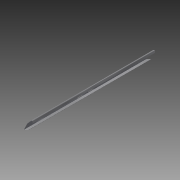
# Autodesk Inventor part: 2in rail right
Saved by Autodesk Inventor 2015 SP1 (Build 190203100, 203)
## iProperties
Created: 2015-01-12
Part Number: 2in rail right
Material: Steel, Alloy
Document SubType Name: Modeling
Designer: Jarod
Density: 7.73 g/cm^3
Appearance: Semi-Polished
Author: Jarod
Autodesk Inventor part; units mm, degrees
ref_plane "YZ Plane" through (0, 0, 0) normal (1, 0, 0) x (0, 1, 0)
ref_plane "XZ Plane" through (0, 0, 0) normal (0, 1, 0) x (-1, 0, 0)
ref_plane "XY Plane" through (0, 0, 0) normal (0, 0, 1) x (1, 0, 0)
sketch "Sketch1" plane through (0, 0, 0) normal (0, 0, 1) x (1, 0, 0)
  line L0 (0, 0) -> (-12.7, 0) construction
  line L1 (-12.7, 0) -> (-12.7, 53.975) construction
  line L2 (-12.7, 53.975) -> (0, 53.975) construction
  line L3 (0, 53.975) -> (0, 0) construction
  line L4 (-12.7, 53.975) -> (-25.4, 53.975) construction
  line L5 (-12.7, 53.975) -> (0, 53.975) construction
  line L6 (-25.4, 53.975) -> (-25.4, 0) construction
  line L7 (-25.4, 0) -> (-12.7, 0) construction
  circle A0 centre (-12.7, 6.35) radius 6.35 construction
  circle A1 centre (-12.7, 47.625) radius 6.35 construction
  line L8 (-12.7, 47.625) -> (-18.1993, 50.8) construction
  line L9 (-12.7, 47.625) -> (-6.35, 47.625) construction
  line L10 (-12.7, 47.625) -> (-7.2007, 50.8) construction
  line L11 (-12.7, 47.625) -> (-6.35, 47.625) construction
  line L12 (0, 0) -> (-25.4, 0)
  line L13 (0, 0) -> (0, -1.5875)
  line L14 (0, 0) -> (1.5875, 0) construction
  line L15 (0, -1.5875) -> (-26.9875, -1.5875)
  arc A2 (-7.2007, 50.8) -> (-18.1993, 50.8) centre (-12.7, 47.625) ccw
  line L16 (-7.2007, 50.8) -> (0, 38.328)
  line L17 (-7.2007, 50.8) -> (7.2007, 50.8) construction
  line L18 (-18.1993, 50.8) -> (-24.5493, 39.8015)
  line L19 (-18.1993, 50.8) -> (-5.4993, 50.8) construction
  line L20 (-25.4, 0) -> (-25.4, 36.6265)
  line L21 (-19.5741, 51.5937) -> (-26.1368, 40.2268)
  line L22 (-26.9875, -1.5875) -> (-26.9875, 37.0518)
  arc A3 (-26.1368, 40.2268) -> (-26.9875, 37.0518) centre (-20.6375, 37.0518) ccw
  arc A4 (-24.5493, 39.8015) -> (-25.4, 36.6265) centre (-19.05, 36.6265) ccw
  line L23 (-5.8259, 51.5937) -> (1.3748, 39.1217)
  arc A5 (-5.8259, 51.5937) -> (-19.5741, 51.5937) centre (-12.7, 47.625) ccw
  arc A6 (0, 38.328) -> (1.3748, 39.1217) centre (0.6874, 38.7248) ccw
  point P0 (-25.4, 38.328)
  dimension "d0" = 12.7
  dimension "d1" = 53.975
  dimension "d2" = 12.7
  dimension "d3" = 180
  dimension "d4" = 53.975
  dimension "d5" = 90
  dimension "d6" = 12.7
  dimension "d7" = 12.7
  dimension "d8" = 6.35
  dimension "d9" = 6.35
  dimension "d10" = 6.35
  dimension "d11" = 150
  dimension "d12" = 6.35
  dimension "d13" = 30
  dimension "d14" = 1.5875
  dimension "d15" = 90
  dimension "d16" = 26.9875
  dimension "d17" = 6.35
  dimension "d18" = 60
  dimension "d19" = 120
  dimension "d20" = 90
  dimension "d21" = 1.5875
  dimension "d22" = 6.35
  dimension "d23" = 6.35
  dimension "d24" = 1.5875
  dimension "d25" = 7.9375
  dimension "d26" = 0
  constraints: 48 end point, 10 point on circle, 8 horizontal, 7 centre point, 6 equal length, 6 point on line, 6 tangent, 4 parallel, 3 perpendicular, 2 vertical
  measures "d0" distance of L1.end L2.end
  measures "d1" distance of L0.end L1.end
  measures "d2" distance of L1.end L4.end
  measures "d3" angle of L4 L5
  measures "d4" distance of L4.end L6.end
  measures "d5" angle of L6 L4
  measures "d6" diameter of A0
  measures "d7" diameter of A1
  measures "d8" distance from line of L0 A0.centre
  measures "d9" distance from line of L2 L8.start
  measures "d10" distance of L8.start L8.end
  measures "d11" angle of L9 L8
  measures "d12" distance of L8.start L10.end
  measures "d13" angle of L11 L10
  measures "d14" distance of L0.start L13.end
  measures "d15" angle of L13 L14
  measures "d16" distance of L13.end L15.end
  measures "d17" radius of A2
  measures "d18" angle of L16 L17
  measures "d19" angle of L18 L19
  measures "d20" angle of L15 L22
  measures "d21" distance between parallel lines of L21 L18
  measures "d22" radius of A3
  measures "d23" radius of A4
  measures "d24" distance between parallel lines of L16 L23
  measures "d25" radius of A5
  measures "d26" distance of L8.start A5.centre
extrude "Extrusion1" add sketch "Sketch1" along normal blind 1689.1
sketch "Sketch2" plane through (-26.9875, -1.5875, 0) normal (-1, 0, 0) x (0, 0, 1)
  line L0 (0, 38.6393) -> (0, 0) projected
  line L1 (0, 0) -> (1689.1, 0) projected
  line L2 (1689.1, 38.6393) -> (1689.1, 0) projected
  line L3 (0, 38.6393) -> (1689.1, 38.6393) projected
  point P0 (0, 1.5875)
  point P1 (1651, 19.05)
  dimension "d29" = 19.05
  dimension "d30" = 38.1
  measures "d29" distance from line of point (1651, 19.05) L1
  measures "d30" distance from line of point (1651, 19.05) L2
hole "Hole1" at (-26.9875, 17.4625, 1651) direction (1, 0, 0) diameter 9.525 end through all
sketch "Sketch3" plane through (-26.9875, -1.5875, 0) normal (-1, 0, 0) x (0, 0, 1)
  circle A0 centre (1651, 19.05) radius 4.7625 projected
  line L0 (0, 38.6393) -> (0, 0) projected
  line L1 (0, 0) -> (1689.1, 0) projected
  line L2 (1689.1, 38.6393) -> (1689.1, 0) projected
  line L3 (0, 38.6393) -> (1689.1, 38.6393) projected
  circle A1 centre (31.75, 19.05) radius 4.7625
  line L4 (15.875, 28.575) -> (15.875, 25.4) construction
  line L5 (15.875, 28.575) -> (15.875, 31.75) construction
  line L6 (12.7, 28.575) -> (12.7, 31.75) construction
  line L7 (12.7, 28.575) -> (12.7, 25.4) construction
  line L8 (15.875, 12.7) -> (15.875, 15.875) construction
  line L9 (12.7, 12.7) -> (12.7, 15.875) construction
  line L10 (15.875, 12.7) -> (15.875, 9.525) construction
  line L11 (12.7, 12.7) -> (12.7, 9.525) construction
  arc A2 (15.875, 25.4) -> (15.875, 31.75) centre (15.875, 28.575) ccw
  arc A3 (12.7, 31.75) -> (12.7, 25.4) centre (12.7, 28.575) ccw
  arc A4 (15.875, 9.525) -> (15.875, 15.875) centre (15.875, 12.7) ccw
  arc A5 (12.7, 15.875) -> (12.7, 9.525) centre (12.7, 12.7) ccw
  line L12 (15.875, 31.75) -> (12.7, 31.75)
  line L13 (15.875, 25.4) -> (12.7, 25.4)
  line L14 (15.875, 15.875) -> (12.7, 15.875)
  line L15 (15.875, 9.525) -> (12.7, 9.525)
  point P0 (0, 1.5875)
  dimension "d45" = 12.7
  dimension "d46" = 15.875
  dimension "d47" = 31.75
  dimension "d48" = 12.7
  dimension "d49" = 15.875
  dimension "d50" = 9.525
  dimension "d51" = 19.05
  dimension "d52" = 12.7
  dimension "d53" = 12.7
  dimension "d54" = 28.575
  dimension "d55" = 28.575
  dimension "d56" = 3.175
  dimension "d57" = 3.175
  dimension "d58" = 3.175
  dimension "d59" = 3.175
  dimension "d60" = 3.175
  dimension "d61" = 3.175
  dimension "d62" = 3.175
  dimension "d63" = 3.175
  dimension "d64" = 3.175
  dimension "d65" = 3.175
  dimension "d66" = 3.175
  dimension "d67" = 3.175
  constraints: 24 end point, 8 point on circle, 8 vertical, 5 centre point, 1 coincident
  measures "d45" distance from line of L0 L6.start
  measures "d46" distance from line of L0 L4.start
  measures "d47" distance from line of L0 point (31.75, 19.05)
  measures "d48" distance from line of L0 L9.start
  measures "d49" distance from line of L0 L8.start
  measures "d50" diameter of A1
  measures "d51" distance from line of L1 A1.centre
  measures "d52" distance from line of L9.start L1
  measures "d53" distance from line of L1 L8.start
  measures "d54" distance from line of L6.start L1
  measures "d55" distance from line of L4.start L1
  measures "d56" distance of L4.start L4.end
  measures "d57" distance of L4.start L5.end
  measures "d58" distance of L6.start L6.end
  measures "d59" distance of L6.start L7.end
  measures "d60" distance of L8.start L8.end
  measures "d61" distance of L9.start L9.end
  measures "d62" distance of L8.start L10.end
  measures "d63" distance of L9.start L11.end
  measures "d64" radius of A2
  measures "d65" radius of A3
  measures "d66" radius of A4
  measures "d67" radius of A5
extrude "Extrusion2" cut sketch "Sketch3" against normal blind 25.4 contours A1 | L13 A3 L12 A2 | L15 A5 L14 A4
sketch "Sketch4" plane through (-26.9875, -1.5875, 0) normal (-1, 0, 0) x (0, 0, 1)
  line L0 (12.7, 15.875) -> (15.875, 15.875) projected
  arc A0 (15.875, 9.525) -> (15.875, 15.875) centre (15.875, 12.7) ccw projected
  line L1 (15.875, 9.525) -> (12.7, 9.525) projected
  arc A1 (12.7, 15.875) -> (12.7, 9.525) centre (12.7, 12.7) ccw projected
  line L2 (12.7, 31.75) -> (15.875, 31.75) projected
  arc A2 (15.875, 25.4) -> (15.875, 31.75) centre (15.875, 28.575) ccw projected
  line L3 (15.875, 25.4) -> (12.7, 25.4) projected
  arc A3 (12.7, 31.75) -> (12.7, 25.4) centre (12.7, 28.575) ccw projected
  circle A4 centre (31.75, 19.05) radius 4.7625 projected
  circle A5 centre (1651, 19.05) radius 4.7625 projected
  line L4 (0, 38.6393) -> (0, 0) projected
  line L5 (0, 0) -> (1689.1, 0) projected
  line L6 (1689.1, 38.6393) -> (1689.1, 0) projected
  line L7 (0, 38.6393) -> (1689.1, 38.6393) projected
  point P0 (0, 1.5875)
  point P1 (101.6, 25.4)
  point P2 (88.9, 12.7)
  point P3 (76.2, 25.4)
  point P4 (63.5, 12.7)
  dimension "d70" = 63.5
  dimension "d71" = 76.2
  dimension "d72" = 88.9
  dimension "d73" = 101.6
  dimension "d74" = 12.7
  dimension "d77" = 12.7
  dimension "d120" = 25.4
  dimension "d121" = 25.4
  measures "d70" distance from line of L4 point (63.5, 12.7)
  measures "d71" distance from line of L4 point (76.2, 25.4)
  measures "d72" distance from line of L4 point (88.9, 12.7)
  measures "d73" distance from line of L4 point (101.6, 25.4)
  measures "d74" distance from line of L5 point (63.5, 12.7)
  measures "d77" distance from line of L5 point (88.9, 12.7)
  measures "d120" distance from line of point (76.2, 25.4) L5
  measures "d121" distance from line of L5 point (101.6, 25.4)
hole "Hole2" at (-26.9875, 23.8125, 101.6) at (-26.9875, 11.1125, 88.9) at (-26.9875, 23.8125, 76.2) at (-26.9875, 11.1125, 63.5) direction (1, 0, 0) diameter 6.35 end through all
sketch "Sketch6" plane through (-26.9875, -1.5875, 0) normal (-1, 0, 0) x (0, 0, 1)
  circle A0 centre (76.2, 25.4) radius 3.175 projected
  circle A1 centre (101.6, 25.4) radius 3.175 projected
  circle A2 centre (88.9, 12.7) radius 3.175 projected
  circle A3 centre (63.5, 12.7) radius 3.175 projected
  line L0 (12.7, 15.875) -> (15.875, 15.875) projected
  arc A4 (15.875, 9.525) -> (15.875, 15.875) centre (15.875, 12.7) ccw projected
  line L1 (15.875, 9.525) -> (12.7, 9.525) projected
  arc A5 (12.7, 15.875) -> (12.7, 9.525) centre (12.7, 12.7) ccw projected
  line L2 (12.7, 31.75) -> (15.875, 31.75) projected
  arc A6 (15.875, 25.4) -> (15.875, 31.75) centre (15.875, 28.575) ccw projected
  line L3 (15.875, 25.4) -> (12.7, 25.4) projected
  arc A7 (12.7, 31.75) -> (12.7, 25.4) centre (12.7, 28.575) ccw projected
  circle A8 centre (31.75, 19.05) radius 4.7625 projected
  circle A9 centre (1651, 19.05) radius 4.7625 projected
  line L4 (0, 38.6393) -> (0, 0) projected
  line L5 (0, 0) -> (1689.1, 0) projected
  line L6 (1689.1, 38.6393) -> (1689.1, 0) projected
  line L7 (0, 38.6393) -> (1689.1, 38.6393) projected
  line L8 (787.4, 6.35) -> (838.2, 6.35)
  line L9 (838.2, 6.35) -> (838.2, 31.75)
  line L10 (838.2, 31.75) -> (787.4, 31.75)
  line L11 (787.4, 31.75) -> (787.4, 6.35)
  line L12 (901.7, 6.35) -> (952.5, 6.35)
  line L13 (952.5, 6.35) -> (952.5, 31.75)
  line L14 (952.5, 31.75) -> (901.7, 31.75)
  line L15 (901.7, 31.75) -> (901.7, 6.35)
  point P0 (0, 1.5875)
  dimension "d98" = 50.8
  dimension "d99" = 25.4
  dimension "d100" = 50.8
  dimension "d101" = 25.4
  dimension "d102" = 787.4
  dimension "d103" = 901.7
  dimension "d104" = 6.35
  dimension "d105" = 6.35
  constraints: 16 end point, 4 parallel, 2 horizontal, 2 perpendicular
  measures "d98" distance of L10.end L9.end
  measures "d99" distance of L9.end L8.end
  measures "d100" distance of L14.end L13.end
  measures "d101" distance of L13.end L12.end
  measures "d102" distance between parallel lines of L4 L11
  measures "d103" distance between parallel lines of L4 L15
  measures "d104" distance between parallel lines of L5 L12
  measures "d105" distance between parallel lines of L5 L8
extrude "Extrusion3" cut sketch "Sketch6" against normal blind 25.4 contours L11 L10 L9 L8 | L15 L14 L13 L12
sketch "Sketch8" plane through (-26.9875, -1.5875, 0) normal (-1, 0, 0) x (0, 0, 1)
  line L0 (838.2, 31.75) -> (838.2, 6.35) projected
  line L1 (838.2, 6.35) -> (787.4, 6.35) projected
  line L2 (787.4, 6.35) -> (787.4, 31.75) projected
  line L3 (787.4, 31.75) -> (838.2, 31.75) projected
  line L4 (952.5, 31.75) -> (952.5, 6.35) projected
  line L5 (952.5, 6.35) -> (901.7, 6.35) projected
  line L6 (901.7, 6.35) -> (901.7, 31.75) projected
  line L7 (901.7, 31.75) -> (952.5, 31.75) projected
  circle A0 centre (76.2, 25.4) radius 3.175 projected
  circle A1 centre (101.6, 25.4) radius 3.175 projected
  circle A2 centre (88.9, 12.7) radius 3.175 projected
  circle A3 centre (63.5, 12.7) radius 3.175 projected
  line L8 (12.7, 15.875) -> (15.875, 15.875) projected
  arc A4 (15.875, 9.525) -> (15.875, 15.875) centre (15.875, 12.7) ccw projected
  line L9 (15.875, 9.525) -> (12.7, 9.525) projected
  arc A5 (12.7, 15.875) -> (12.7, 9.525) centre (12.7, 12.7) ccw projected
  line L10 (12.7, 31.75) -> (15.875, 31.75) projected
  arc A6 (15.875, 25.4) -> (15.875, 31.75) centre (15.875, 28.575) ccw projected
  line L11 (15.875, 25.4) -> (12.7, 25.4) projected
  arc A7 (12.7, 31.75) -> (12.7, 25.4) centre (12.7, 28.575) ccw projected
  circle A8 centre (31.75, 19.05) radius 4.7625 projected
  circle A9 centre (1651, 19.05) radius 4.7625 projected
  line L12 (0, 38.6393) -> (0, 0) projected
  line L13 (0, 0) -> (1689.1, 0) projected
  line L14 (1689.1, 38.6393) -> (1689.1, 0) projected
  line L15 (0, 38.6393) -> (1689.1, 38.6393) projected
  point P0 (0, 1.5875)
  point P1 (965.2, 19.05)
  point P2 (774.7, 19.05)
  dimension "d122" = 19.05
  dimension "d123" = 19.05
  dimension "d124" = 190.5
  dimension "d125" = 774.7
  measures "d122" distance from line of L13 point (965.2, 19.05)
  measures "d123" distance from line of L13 point (774.7, 19.05)
  measures "d124" distance of point (965.2, 19.05) point (774.7, 19.05)
  measures "d125" distance from line of L12 point (774.7, 19.05)
hole "Hole5" at (-26.9875, 17.4625, 965.2) at (-26.9875, 17.4625, 774.7) direction (1, 0, 0) diameter 6.35 end through all
sketch "Sketch9" plane through (0, -1.5875, 0) normal (0, -1, 0) x (1, 0, 0)
  line L0 (-26.9875, 0) -> (0, 0) projected
  line L1 (0, 0) -> (0, 1689.1) projected
  line L2 (-26.9875, 1689.1) -> (0, 1689.1) projected
  point P0 (-12.7, 25.4)
  point P1 (-12.7, 1676.4)
  dimension "d135" = 12.7
  dimension "d136" = 12.7
  dimension "d137" = 12.7
  dimension "d138" = 25.4
  measures "d135" distance from line of L1 point (-12.7, 1676.4)
  measures "d136" distance from line of L2 point (-12.7, 1676.4)
  measures "d137" distance from line of L1 point (-12.7, 25.4)
  measures "d138" distance from line of L0 point (-12.7, 25.4)
hole "Hole6" at (-12.7, -1.5875, 25.4) at (-12.7, -1.5875, 1676.4) direction (0, 1, 0) diameter 6.35 depth 25.4 tip angle 118
sketch "Sketch10" plane through (0, 0, 1689.1) normal (0, 0, 1) x (1, 0, 0)
  line L0 (0, 0) -> (-25.4, 0) projected
  line L1 (-25.4, 0) -> (-25.4, 36.6265) projected
  arc A0 (-24.5493, 39.8015) -> (-25.4, 36.6265) centre (-19.05, 36.6265) ccw projected
  line L2 (-24.5493, 39.8015) -> (-18.1993, 50.8) projected
  arc A1 (-7.2007, 50.8) -> (-18.1993, 50.8) centre (-12.7, 47.625) ccw projected
  line L3 (-7.2007, 50.8) -> (0, 38.328) projected
  arc A2 (0, 38.328) -> (1.3748, 39.1217) centre (0.6874, 38.7248) ccw projected
  line L4 (1.3748, 39.1217) -> (-5.8259, 51.5937) projected
  arc A3 (-5.8259, 51.5937) -> (-19.5741, 51.5937) centre (-12.7, 47.625) ccw projected
  line L5 (-19.5741, 51.5937) -> (-26.1368, 40.2268) projected
  arc A4 (-26.1368, 40.2268) -> (-26.9875, 37.0518) centre (-20.6375, 37.0518) ccw projected
  line L6 (-26.9875, 37.0518) -> (-26.9875, -1.5875) projected
  line L7 (-26.9875, -1.5875) -> (0, -1.5875) projected
  line L8 (0, -1.5875) -> (0, 0) projected
extrude "Extrusion4" cut sketch "Sketch10" against normal blind 19.05
body "Solid1"
